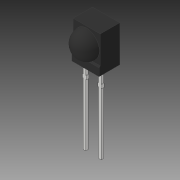
# Autodesk Inventor part: Fotodiode BPV23F
Saved by Autodesk Inventor 2017.3 (Build 213256000, 256)
## iProperties
Part Number: Fotodiode BPV23F
Material: Generisch
Document SubType Name: Modeling
Designer: rYan
Density: 1 g/cm^3
Appearance: Vorgabe
Author: rYan
Autodesk Inventor part; units mm, degrees
ref_plane "YZ Plane" through (0, 0, 0) normal (1, 0, 0) x (0, 1, 0)
ref_plane "XZ Plane" through (0, 0, 0) normal (0, 1, 0) x (-1, 0, 0)
sketch "Skizze3" plane through (0, 0, 0) normal (1, 0, 0) x (0, 1, 0)
  line L0 (3.2, 2.5) -> (0, 2.5)
  line L1 (0, 2.5) -> (0, -2.05)
  line L2 (0, -2.05) -> (-0.2, -2.25)
  line L3 (-0.2, -2.25) -> (-0.2, -3.5)
  line L4 (-0.2, -3.5) -> (3.2, -3.5)
  line L5 (3.2, -3.5) -> (3.2, 2.5)
  line L6 (0, 3.7) -> (0, -4.7) projected
  line L7 (-0.88, 0) -> (3.88, 0) projected
  point P0 (0, 0)
  dimension "d5" = 3.2
  dimension "d6" = 6
  dimension "d7" = 2.5
  dimension "d8" = 3.4
  dimension "d9" = 45
  dimension "d10" = 4.55
  constraints: 12 end point, 3 perpendicular, 1 collinear, 1 horizontal, 1 parallel
  measures "d5" distance of L0.start L0.end
  measures "d6" distance of L4.end L0.start
  measures "d7" distance between parallel lines of L7 L0
  measures "d8" distance of L3.end L4.end
  measures "d9" angle of L2 L3
  measures "d10" distance of L0.end L1.end
extrude "Extrusion2" add sketch "Skizze3" along normal mid plane 4.5
sketch "Skizze4" plane through (0, 0, 0) normal (1, 0, 0) x (0, 1, 0)
  line L0 (0, -2.05) -> (0, 2.5) projected
  arc A0 (0, 2.245) -> (0, -2.245) centre (0.15, 0) ccw
  line L1 (3.2, 2.5) -> (0, 2.5) projected
  line L2 (0, 2.245) -> (0, -2.245)
  point P0 (0, 0)
  dimension "d13" = 2.25
  dimension "d14" = 0.15
  dimension "d15" = 2.5
  constraints: 2 end point, 2 point on circle, 2 point on line, 1 centre point, 1 vertical
  measures "d13" radius of A0
  measures "d14" distance from line of A0.centre L0
  measures "d15" distance from line of L1 A0.centre
revolve "Umdrehung1" add sketch "Skizze4" angle 180 mid plane about axis through (0, 0, -2.05) along (0, 0, 1)
ref_plane "Arbeitsebene1" through (-2.25, 0.9, -3.5) normal (0, -1, 0) x (1, 0, 0)
sketch "Skizze5" plane through (-2.25, 0.9, -3.5) normal (0, -1, 0) x (1, 0, 0)
  line L0 (0.755, 0) -> (1.205, 0)
  line L1 (1.205, -12.8) -> (0.755, -12.8)
  line L2 (0, 0) -> (4.5, 0) projected
  line L3 (1.305, -2) -> (1.305, -2.6)
  line L4 (0.655, -2.6) -> (0.655, -2)
  line L5 (0.655, -2) -> (0.755, -2)
  line L6 (1.205, -2) -> (1.305, -2)
  line L7 (1.305, -2.6) -> (1.205, -2.6)
  line L8 (0.755, -2.6) -> (0.655, -2.6)
  line L9 (0.755, -12.8) -> (0.755, -2.6)
  line L10 (0.755, -2) -> (0.755, 0)
  line L11 (1.205, 0) -> (1.205, -2)
  line L12 (1.205, -2.6) -> (1.205, -12.8)
  line L13 (0.98, -12.8) -> (0.98, 0) construction
  line L14 (4.5, 6) -> (0, 6) construction
  point P0 (2.25, 3.5)
  dimension "d18" = 0.45
  dimension "d19" = 0.65
  dimension "d20" = 0.6
  dimension "d21" = 8.6
  dimension "d22" = 18.8
  dimension "d23" = 1.27
  constraints: 26 end point, 10 parallel, 5 perpendicular, 3 collinear, 3 horizontal, 1 midpoint, 1 point on line, 3 other
  measures "d18" distance between parallel lines of L10 L11
  measures "d19" distance between parallel lines of L4 L3
  measures "d20" distance of L3.start L3.end
  measures "d21" distance between parallel lines of L14 L7
  measures "d22" distance between parallel lines of L14 L1
  measures "d23" distance from line of point (2.25, 3.5) L13
extrude "Extrusion3" add sketch "Skizze5" against normal blind 0.4
mirror "Spiegeln1" about plane through (0, 0, 0) normal (1, 0, 0) of "Extrusion3"
